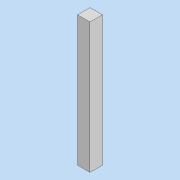
# Autodesk Inventor part: loadstick
Saved by Autodesk Inventor 2022 (Build 260153000, 153)
## iProperties
Created: 2024-05-21
Part Number: loadstick
Material: 一般
Document SubType Name: Modeling
Designer: ktamu
Density: 1 g/cm^3
Appearance: 既定
Mass: 0.672 g
Surface Area: 7.04 cm^2
Volume: 0.672 cm^3
Author: ktamu
Autodesk Inventor part; units mm, degrees
ref_plane "YZ Plane" through (0, 0, 0) normal (1, 0, 0) x (0, 1, 0)
ref_plane "XZ Plane" through (0, 0, 0) normal (0, 1, 0) x (-1, 0, 0)
ref_plane "XY Plane" through (0, 0, 0) normal (0, 0, 1) x (1, 0, 0)
sketch "スケッチ1" plane through (0, 0, 0) normal (0, 0, 1) x (1, 0, 0)
  point P0 (0, 0)
sketch "スケッチ2" plane through (0, 0, 0) normal (0, 1, 0) x (-1, 0, 0)
  line L0 (2, 2) -> (-2, 2)
  line L1 (-2, 2) -> (-2, -2)
  line L2 (-2, -2) -> (2, -2)
  line L3 (2, -2) -> (2, 2)
  line L4 (2, 2) -> (-2, -2) construction
  line L5 (-2, 2) -> (2, -2) construction
  point P0 (0, 0)
  dimension "d0" = 4
  dimension "d1" = 4
  constraints: 12 end point, 2 midpoint, 2 parallel, 1 horizontal, 1 perpendicular
  measures "d0" distance of L2.end L1.end
  measures "d1" distance of L1.end L0.end
extrude "押し出し1" add sketch "スケッチ2" along normal mid plane 42
